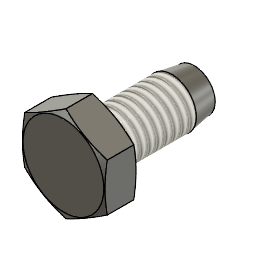
Elektrikli scooter (Autodesk Fusion 360 archive; units mm, degrees)
design "Düz Normal Altıgen Başlı Kılavuz Vida ANSI B18.6.4 10-32 UNF x 0.375 Tip C Çelik Sınıf 2 Düz"
description: Düz Normal Altıgen Başlı Kılavuz Vida ANSI B18.6.4 10-32 UNF x 0.375 Tip C
part number: PRHHTSTC ANSI B18.6.4 - 10-32 UNF x 0.375 Çelik Sınıf 2 Düz
Autodesk Fusion 360 part; units mm, degrees
sketch "Sketch1" plane through (0, 0, 0) normal (0, 1, 0) x (1, 0, 0)
  line L0 (-2.413, 0) -> (-2.413, 9.525)
  line L1 (-2.413, 9.525) -> (0, 9.525)
  line L2 (0, 9.525) -> (0, -3.048)
  line L3 (-2.413, 0) -> (-3.8832, 0)
  line L4 (-4.5766, -0.2524) -> (-4.5766, -2.7956)
  line L5 (-3.8832, -3.048) -> (0, -3.048)
  line L6 (-3.8832, 0) -> (-4.5766, -0.2524)
  line L7 (-3.8832, -3.048) -> (-4.5766, -2.7956)
  dimension "d9" = 4.826
  dimension "d111" = 3.048
  dimension "d112" = 20
  dimension "d113" = 20
  dimension "d114" = 9.1531
  dimension "d156" = 7.7663
  dimension "d165" = 9.525
  constraint perpendicular L0 L1
  constraint collinear origin L1.end L2.end
  constraint perpendicular L0 L3
  constraint coincident origin L3
  constraint vertical L0
  constraint vertical L2
  constraint coincident L2 L5.end
  constraint vertical L5.start L3.end
  measures "d111" distance of L3 L5
  measures "d112" angle of L3 L6
  measures "d113" angle of L5 L7
  measures "d165" distance of origin L1
revolve "Revolve1" add sketch "Sketch1" angle 360 about axis through (0, 0, -9.525) along (0, 0, 1)
sketch "Sketch8" plane through (0, 0, 0) normal (0, 0, 1) x (1, 0, 0)
  circle A0 centre (0, 0) radius 4.5766
  line L0 (-3.9634, -2.2883) -> (0, -4.5766)
  line L1 (0, -4.5766) -> (3.9634, -2.2883)
  line L2 (3.9634, -2.2883) -> (3.9634, 2.2883)
  line L3 (3.9634, 2.2883) -> (0, 4.5766)
  line L4 (0, 4.5766) -> (-3.9634, 2.2883)
  line L5 (-3.9634, 2.2883) -> (-3.9634, -2.2883)
  constraint coincident A0.centre origin
  constraint coincident A0 L0.start
  constraint vertical L5
extrude "Extrude5" cut sketch "Sketch8" along normal blind 3.048 contours A0 L2 | A0 L3 | A0 L1 | A0 L4 | A0 L0 | A0 L5
thread "Thread1" "ANSI Unified Screw Threads 0.19(#10) 10-32 UNF 10-32 UNF 2A" major diameter 4.7269 minor diameter 3.8583 pitch 0.7937 angle 60 resizes the face on face at (-2.401, 0.2403, -3.175)
sketch "Sketch5" plane through (0, 0, 0) normal (0, 1, 0) x (1, 0, 0)
  line L0 (-2.4613, 9.525) -> (-2.4613, 6.7564)
  line L1 (-2.4613, 6.7564) -> (-2.0066, 9.525)
  line L2 (0, 9.525) -> (0, -3.048)
  line L3 (-2.4613, 9.525) -> (0, 9.525)
  dimension "d162" = 2.7686
  dimension "d163" = 2.0066
  dimension "d164" = 2.4613
  constraint coincident L2.start L3.end
  constraint perpendicular L2 L3
  constraint coincident L1.end L3
  constraint perpendicular L0 L3
  measures "d162" distance of L0.end L3
  measures "d163" distance of L1.end L2
  measures "d164" distance of L0 L2.start
revolve "Revolve2" cut sketch "Sketch5" angle 360 about axis through (0, 0, -9.525) along (0, 0, 1)
equation "d9 = adsk_nomdia"
equation "d89 = adsk_headh"
equation "d111 = adsk_headh"
equation "d112 = adsk_chamang1"
equation "d113 = adsk_chamang2"
equation "d114 = adsk_headdia"
equation "adsk_nomlen = 0.375 in"
equation "adsk_headh = 0.12 in"
equation "adsk_nomdia = 0.19 in"
equation "adsk_waflat = 0.312 in"
equation "adsk_startlen = 0.109 in"
equation "adsk_endpointdia = 0.158 in"
equation "adsk_beardia = adsk_waflat * 0.98"
equation "d156 = adsk_beardia"
equation "adsk_headdia = 0.36036 in"
equation "adsk_chamang1 = 20 deg"
equation "adsk_chamang2 = 20 deg"
equation "d162 = adsk_startlen"
equation "d163 = adsk_endpointdia / 2"
equation "d164 = adsk_nomdia * 0.51"
equation "d165 = adsk_nomlen"

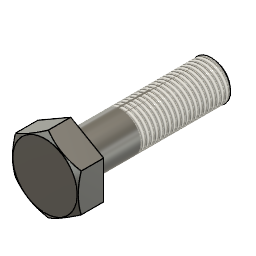
design "Ağır Altıgen Cıvata ANSI B18.2.3.6M - M36 x 4 x 130 Çelik Sınıf 2 Düz"
description: Ağır Altıgen Cıvata ANSI B18.2.3.6M - M36 x 4 x 130
part number: HHB ANSI B18.2.3.6M - M36 x 4 x 130 Çelik Sınıf 2 Düz
Autodesk Fusion 360 part; units mm, degrees
sketch "Sketch1" plane through (0, 0, 0) normal (0, 1, 0) x (1, 0, 0)
  line L0 (-18, 0) -> (-18, 130)
  line L1 (-18, 130) -> (0, 130)
  line L2 (0, 130) -> (0, -23.55)
  line L3 (-18, 0) -> (-34.65, 0)
  line L4 (-34.65, 0) -> (-34.65, -20.5189)
  line L5 (-29.4, -23.55) -> (0, -23.55)
  line L6 (-34.65, -20.5189) -> (-29.4, -23.55)
  dimension "d81" = 69.3
  dimension "d135" = 36
  dimension "d139" = 23.55
  dimension "d140" = 130
  dimension "d156" = 58.8
  dimension "d158" = 30
  constraint perpendicular L0 L1
  constraint collinear origin L1.end L2.end
  constraint perpendicular L0 L3
  constraint coincident origin L3
  constraint vertical L2
  constraint coincident L2 L5.end
  constraint coincident L0.start L3.start
  constraint coincident L0.end L1.start
  constraint vertical L4
  measures "d139" distance of L3 L5
  measures "d140" distance of L1 L3
  measures "d158" angle of L5 L6
revolve "Revolve1" add sketch "Sketch1" angle 360 about axis through (0, 0, -130) along (0, 0, 1)
sketch "Sketch8" plane through (0, 0, 23.55) normal (0, 0, 1) x (1, 0, 0)
  circle A0 centre (0, 0) radius 34.65
  line L0 (-30.0078, -17.325) -> (0, -34.65)
  line L1 (0, -34.65) -> (30.0078, -17.325)
  line L2 (30.0078, -17.325) -> (30.0078, 17.325)
  line L3 (30.0078, 17.325) -> (0, 34.65)
  line L4 (0, 34.65) -> (-30.0078, 17.325)
  line L5 (-30.0078, 17.325) -> (-30.0078, -17.325)
  constraint coincident A0 L0.start
  constraint coincident A0.centre origin
  constraint vertical L5
extrude "Extrude5" cut sketch "Sketch8" against normal blind 23.55 contours A0 L2 | A0 L3 | A0 L1 | A0 L4 | A0 L0 | A0 L5
fillet "Fillet7" radius 1 1 edges at (-16.7819, 6.5091, 0)
thread "Thread4" "ANSI Metric M Profile 36.0 M36x4 M36x4 6g" major diameter 35.7025 minor diameter 31.132 pitch 4 angle 60 resizes the face on face at (-17.9106, 1.7922, -87) from (0, 0, -46) to (0, 0, -130)
sketch "Sketch13" plane through (0, 0, 0) normal (0, 1, 0) x (1, 0, 0)
  line L0 (0, 130) -> (0, -23.55) construction
  line L1 (0, 130) -> (-18.36, 130)
  line L2 (-18.36, 130) -> (-18.36, 127.5462)
  line L3 (-18.36, 127.5462) -> (-15.5462, 130)
  dimension "d160" = 2.4538
  dimension "d161" = 15.5462
  dimension "d162" = 18.36
  constraint coincident L0.start L1.start
  constraint perpendicular L0 L1
  constraint perpendicular L1 L2
  constraint coincident L1 L3.end
  measures "d160" distance of L1 L2.end
  measures "d161" distance of L0 L3.end
  measures "d162" distance of L0.start L2
revolve "Revolve4" cut sketch "Sketch13" angle 360 about axis through (0, 0, 1.75) along (0, 0, 1)
equation "adsk_nomlen = 130.00 mm"
equation "adsk_headh = 23.55 mm"
equation "adsk_headdia = 69.30 mm"
equation "adsk_nomdia = 36.00 mm"
equation "d81 = adsk_headdia"
equation "d89 = -adsk_headh"
equation "adsk_waflat = 60.00 mm"
equation "adsk_thrlen = 84.00 mm"
equation "adsk_midfillet = 1.00 mm"
equation "d135 = adsk_nomdia"
equation "d139 = adsk_headh"
equation "d140 = adsk_nomlen"
equation "d142 = adsk_midfillet"
equation "adsk_endpointdia = 31.0924 mm"
equation "adsk_startlen = 2.4538 mm"
equation "d156 = adsk_waflat * 0.98"
equation "d158 = adsk_chamang2"
equation "adsk_chamang2 = 30.00 deg"
equation "d160 = adsk_startlen"
equation "d161 = adsk_endpointdia / 2"
equation "d162 = adsk_nomdia * 0.51"
equation "d166 = min(adsk_thrlen; adsk_nomlen - adsk_midfillet - 0.001 mm)"
